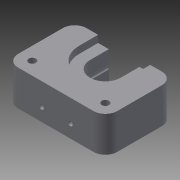
# Autodesk Inventor part: UHMW_block
Saved by Autodesk Inventor 2013 (Build 170138000, 138)
## iProperties
Created: 2013-08-04
Part Number: UHMW_block
Material: Generic
Document SubType Name: Modeling
Designer: employee
Density: 1 g/cm^3
Mass: 14.4379 g
Surface Area: 49.0761 cm^2
Volume: 14.4379 cm^3
Author: employee
Autodesk Inventor part; units mm, degrees
ref_plane "YZ Plane" through (0, 0, 0) normal (1, 0, 0) x (0, 1, 0)
ref_plane "XZ Plane" through (0, 0, 0) normal (0, 1, 0) x (-1, 0, 0)
ref_plane "XY Plane" through (0, 0, 0) normal (0, 0, 1) x (1, 0, 0)
sketch "Sketch1" plane through (0, 0, 0) normal (0, 0, 1) x (1, 0, 0)
  line L0 (-21, 8) -> (21, 8)
  line L1 (21, 8) -> (21, -21)
  line L2 (21, -21) -> (-21, -21)
  line L3 (-21, -21) -> (-21, 8)
  point P0 (0, 0)
  point P1 (0, -21)
  dimension "d0" = 21
  dimension "d1" = 42
  dimension "d2" = 29
  constraints: 8 end point, 2 parallel, 1 horizontal, 1 midpoint, 1 perpendicular, 1 vertical alignment
  measures "d0" distance from line of point (0, 0) L2
  measures "d1" distance of L1.end L2.end
  measures "d2" distance between parallel lines of L0 L2
extrude "Extrusion1" add sketch "Sketch1" along normal blind 15
fillet "Fillet1" radius 5 4 edges at (21, -21, 7.5) (-21, 8, 7.5) (21, 8, 7.5) (-21, -21, 7.5)
sketch "Sketch2" plane through (0, 0, 15) normal (0, 0, 1) x (1, 0, 0)
  line L0 (16, 8) -> (-16, 8) projected
  arc A0 (-11.05, 0) -> (11.05, 0) centre (0, 0) ccw
  line L1 (-11.05, 0) -> (-11.05, 8)
  line L2 (11.05, 0) -> (11.05, 8)
  dimension "d6" = 11.05
  constraints: 4 end point, 2 perpendicular, 2 point on circle, 2 point on line, 2 tangent, 1 centre point, 1 coincident
  measures "d6" radius of A0
extrude "Extrusion2" cut sketch "Sketch2" against normal blind 3
sketch "Sketch3" plane through (0, 0, 12) normal (0, 0, 1) x (1, 0, 0)
  arc A0 (-11.05, 0) -> (11.05, 0) centre (0, 0) ccw projected
  line L0 (-11.05, 8) -> (11.05, 8) projected
  line L1 (-6.5, 8) -> (-6.5, 0)
  arc A1 (-6.5, 0) -> (6.5, 0) centre (0, 0) ccw
  line L2 (6.5, 0) -> (6.5, 8)
  dimension "d10" = 13
  constraints: 4 end point, 2 point on circle, 2 point on line, 2 tangent, 1 centre point, 1 concentric, 1 parallel, 1 perpendicular
  measures "d10" distance between parallel lines of L2 L1
extrude "Extrusion3" cut sketch "Sketch3" against normal through all
sketch "Sketch4" plane through (-16, -21, 0) normal (0, -1, 0) x (1, 0, 0)
  line L0 (32, 0) -> (0, 0) projected
  line L1 (0, 15) -> (32, 15) projected
  line L2 (9.875, 5.5) -> (22.125, 5.5)
  circle A0 centre (9.875, 5.5) radius 1
  circle A1 centre (22.125, 5.5) radius 1
  point P0 (16, 0)
  point P1 (16, 0)
  point P2 (16, 5.5)
  dimension "d14" = 5.5
  dimension "d15" = 12.25
  dimension "d16" = 2
  constraints: 2 centre point, 2 coincident, 2 end point, 2 midpoint, 1 equal radius, 1 parallel, 1 vertical alignment
  measures "d14" distance between parallel lines of L2 L0
  measures "d15" distance of L2.start L2.end
  measures "d16" diameter of A1
extrude "Extrusion4" cut sketch "Sketch4" against normal through all
sketch "Sketch5" plane through (0, 0, 0) normal (0, 0, -1) x (-1, 0, 0)
  arc A0 (-6.5, 0) -> (6.5, 0) centre (0, 0) ccw projected
  line L0 (-15.5, -15.5) -> (-15.5, 15.5)
  line L1 (-15.5, 15.5) -> (15.5, 15.5)
  line L2 (15.5, 15.5) -> (15.5, -15.5)
  line L3 (15.5, -15.5) -> (-15.5, -15.5)
  circle A1 centre (-15.5, -15.5) radius 1.55
  circle A2 centre (15.5, -15.5) radius 1.55
  dimension "d19" = 31
  dimension "d20" = 3.1
  constraints: 8 end point, 3 coincident, 2 centre point, 1 equal radius, 1 horizontal, 9 other
  measures "d19" distance of L2.end L0.start
  measures "d20" diameter of A1
extrude "Extrusion5" cut sketch "Sketch5" against normal through all contours L3 A1 L0 | L0 A1 L3 | A2 L2 L3 | L3 L2 A2
body "Solid1"
